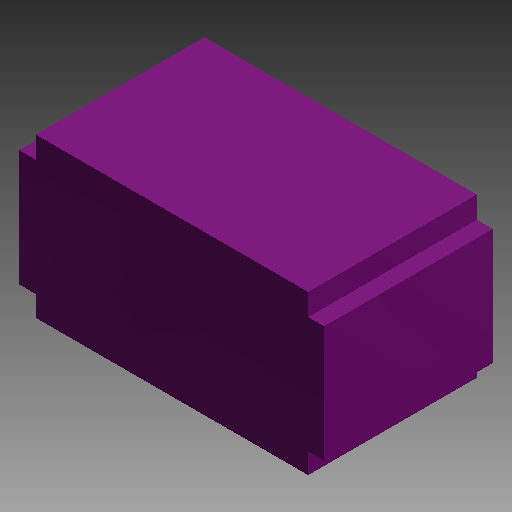
# Autodesk Inventor part: SMAJ30A
Saved by Autodesk Inventor 2018.2 (Build 222227000, 227)
## iProperties
Part Number: SMAJ30A
Material: Generic
Document SubType Name: Modeling
Designer: autocad
Appearance: SMA-SM, SMAJ30A
Author: autocad
Autodesk Inventor part; units mm, degrees
ref_plane "YZ Plane" through (0, 0, 0) normal (1, 0, 0) x (0, 1, 0)
ref_plane "XZ Plane" through (0, 0, 0) normal (0, 1, 0) x (-1, 0, 0)
ref_plane "XY Plane" through (0, 0, 0) normal (0, 0, 1) x (1, 0, 0)
sketch "SMA-SM, SMAJ30A_123" plane through (0, 0, 0) normal (0, 0, 1) x (1, 0, 0)
  line L0 (-2.377, 1.016) -> (-2.377, 1.397)
  line L1 (-2.377, 1.397) -> (2.3876, 1.397)
  line L2 (2.3876, 1.397) -> (2.3876, 1.016)
  line L3 (2.3876, 1.016) -> (2.667, 1.016)
  line L4 (2.667, 1.016) -> (2.667, -1.016)
  line L5 (2.667, -1.016) -> (2.3876, -1.016)
  line L6 (2.3876, -1.016) -> (2.3876, -1.377)
  line L7 (2.3876, -1.377) -> (-2.377, -1.377)
  line L8 (-2.377, -1.377) -> (-2.377, -1.016)
  line L9 (-2.377, -1.016) -> (-2.667, -1.016)
  line L10 (-2.667, -1.016) -> (-2.667, 1.016)
  line L11 (-2.667, 1.016) -> (-2.377, 1.016)
  constraints: 24 end point
extrude "Extrusion1" add sketch "SMA-SM, SMAJ30A_123" along normal blind 2.95
body "Solid1"
